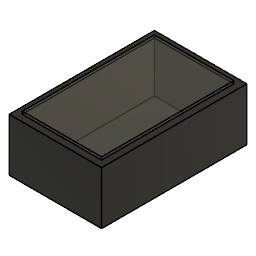
modelo_v1 (Autodesk Fusion 360 design; units mm, degrees)
part number: 2026-04-27-18-00-06-652
Autodesk Fusion 360 part; units mm, degrees
sketch "Boceto1" plane through (0, 0, 0) normal (0, 0, 1) x (1, 0, 0)
  line L0 (0, 0) -> (60, 0)
  line L1 (60, 0) -> (60, 100)
  line L2 (60, 100) -> (0, 100)
  line L3 (0, 100) -> (0, 0)
  line L4 (65, -5) -> (-5, -5)
  line L5 (-5, -5) -> (-5, 105)
  line L6 (-5, 105) -> (65, 105)
  line L7 (65, 105) -> (65, -5)
  line L8 (0, 75) -> (60, 75)
  line L9 (60, 75) -> (60, 100)
  line L10 (60, 100) -> (0, 100)
  line L11 (0, 100) -> (0, 75)
  dimension "d1" = 100
  dimension "d2" = 60
  dimension "d3" = 110
  dimension "d4" = 70
  constraint horizontal L0
  constraint vertical L1
  constraint horizontal L2
  constraint vertical L3
  constraint coincident L0.start L3.end
  constraint perpendicular L3 L4
  constraint perpendicular L4 L5
  constraint perpendicular L5 L6
  constraint perpendicular L4 L7
  constraint horizontal L8
  constraint vertical L9
  constraint horizontal L10
  constraint vertical L11
  constraint coincident L3 L8.start
  measures "d1" distance of L0.start L2.end
  measures "d2" distance of L0.start L0.end
  measures "d3" distance of L4.start L6.end
  measures "d4" distance of L5.end L6.end
extrude "Extruir1" add sketch "Boceto1" along normal blind 40 contours L0 L1 L3 L8 | L1 L2 L3 L8 L9 L10 L11 | L4 L5 L6 L7 makes body 1
sketch "Boceto3" plane through (0, 0, 40) normal (0, 0, 1) x (-1, 0, 0)
  line L0 (-65, -105) -> (5, -105)
  line L1 (5, -105) -> (5, 5)
  line L2 (5, 5) -> (-65, 5)
  line L3 (-65, 5) -> (-65, -105)
  line L4 (-60, 0) -> (-60, -100)
  line L5 (-60, -100) -> (0, -100)
  line L6 (0, -100) -> (0, 0)
  line L7 (0, 0) -> (-60, 0)
  dimension "d8" = -5
extrude "Extruir2" cut sketch "Boceto3" against normal blind 38 contours L4 L5 L6 L7 bodies 1
sketch "Boceto4" plane through (0, 0, 40) normal (0, 0, 1) x (-1, 0, 0)
  line L0 (-60, -100) -> (-60, 0)
  line L1 (-60, 0) -> (0, 0)
  line L2 (0, 0) -> (0, -100)
  line L3 (0, -100) -> (-60, -100)
  line L4 (-65, -105) -> (5, -105)
  line L5 (5, -105) -> (5, 5)
  line L6 (5, 5) -> (-65, 5)
  line L7 (-65, 5) -> (-65, -105)
sketch "Boceto5" plane through (0, 0, 40) normal (0, 0, 1) x (-1, 0, 0)
  line L0 (-60, -100) -> (-60, 0)
  line L1 (-60, 0) -> (0, 0)
  line L2 (0, 0) -> (0, -100)
  line L3 (0, -100) -> (-60, -100)
  line L4 (-65, -105) -> (5, -105)
  line L5 (5, -105) -> (5, 5)
  line L6 (5, 5) -> (-65, 5)
  line L7 (-65, 5) -> (-65, -105)
  line L8 (-30.0059, -70.0059) -> (-29.9941, -70.0059)
  line L9 (-29.9941, -29.9941) -> (-30.0059, -29.9941)
  dimension "d18" = -34.9941
extrude "Extruir6" add sketch "Boceto5" along normal blind 2 separate body contours L0 L1 L2 L3 makes body 2
